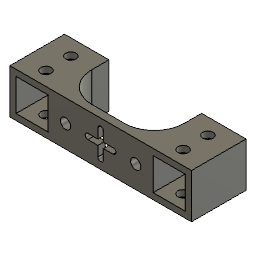
MountingBracket (Autodesk Fusion 360 design; units mm, degrees)
Autodesk Fusion 360 part; units mm, degrees
sketch "Sketch1" plane through (0, 0, 0) normal (0, 0, 1) x (1, 0, 0)
  line L0 (-1.1, 1.1) -> (-1.1, 5.1)
  arc A0 (1.1, 5.1) -> (-1.1, 5.1) centre (0, 5.1) ccw
  line L1 (1.1, 5.1) -> (1.1, 1.1)
  line L2 (-1.1, 5.1) -> (1.1, 5.1) construction
  line L3 (1.1, 1.1) -> (-1.1, 1.1) construction
  line L4 (-1.1, 1.1) -> (-1.1, -1.1) construction
  line L5 (-1.1, -1.1) -> (1.1, -1.1) construction
  line L6 (1.1, -1.1) -> (1.1, 1.1) construction
  line L7 (1.1, 1.1) -> (-1.1, -1.1) construction
  line L8 (-1.1, 1.1) -> (1.1, -1.1) construction
  line L9 (-1.1, -1.1) -> (-5.1, -1.1)
  arc A1 (-5.1, 1.1) -> (-5.1, -1.1) centre (-5.1, 0) ccw
  line L10 (-5.1, 1.1) -> (-1.1, 1.1)
  line L11 (1.1, -1.1) -> (1.1, -5.1)
  arc A2 (-1.1, -5.1) -> (1.1, -5.1) centre (0, -5.1) ccw
  line L12 (-1.1, -5.1) -> (-1.1, -1.1)
  line L13 (1.1, 1.1) -> (5.1, 1.1)
  arc A3 (5.1, -1.1) -> (5.1, 1.1) centre (5.1, 0) ccw
  line L14 (5.1, -1.1) -> (1.1, -1.1)
  line L15 (7.1, 7.1) -> (-7.1, 7.1)
  line L16 (-7.1, 7.1) -> (-7.1, -7.1)
  line L17 (-7.1, -7.1) -> (7.1, -7.1)
  line L18 (7.1, -7.1) -> (7.1, 7.1)
  line L19 (7.1, 7.1) -> (-7.1, -7.1) construction
  line L20 (-7.1, 7.1) -> (7.1, -7.1) construction
  dimension "d2" = 2.2
  dimension "d3" = 2.2
  dimension "d4" = 2.2
  dimension "d5" = 4
  dimension "d7" = 360
  dimension "d37" = 2
  constraint vertical L0
  constraint tangent L0 A0
  constraint vertical L1
  constraint horizontal L2
  constraint horizontal L3
  constraint perpendicular L3 L4
  constraint parallel L3 L5
  constraint parallel L4 L6
  constraint coincident L7 origin
  constraint coincident L8 origin
  constraint coincident L0.start L3.end
  constraint coincident L1.end L3.start
  constraint horizontal L15
  constraint perpendicular L15 L16
  constraint parallel L15 L17
  constraint parallel L16 L18
  constraint coincident L19 origin
  constraint coincident L20 origin
  constraint equal L15 L18
  measures "d2" distance of L0 L1
  measures "d3" distance of L4.end L5.end
  measures "d4" distance of L0.start L4.end
  measures "d5" distance of L2 L3
  measures "d37" distance of A3.centre L18
extrude "Extrude1" add sketch "Sketch1" along normal blind 3
sketch "Sketch2" plane through (0, 0, 0) normal (0, 0, 1) x (1, 0, 0)
  line L0 (-33.9, 6.35) -> (-21.2, 6.35) construction
  line L1 (-21.2, 6.35) -> (-21.2, -6.35) construction
  line L2 (-21.2, -6.35) -> (-33.9, -6.35) construction
  line L3 (-33.9, -6.35) -> (-33.9, 6.35) construction
  line L4 (21.2, 6.35) -> (33.9, 6.35) construction
  line L5 (33.9, 6.35) -> (33.9, -6.35) construction
  line L6 (33.9, -6.35) -> (21.2, -6.35) construction
  line L7 (21.2, -6.35) -> (21.2, 6.35) construction
  line L8 (-21.2, 0) -> (21.2, 0) construction
  line L9 (-21.1, -6.45) -> (-34, -6.45)
  line L10 (-34, -6.45) -> (-34, 6.45)
  line L11 (-34, 6.45) -> (-21.1, 6.45)
  line L12 (-21.1, 6.45) -> (-21.1, -6.45)
  line L13 (-18.6, -8.95) -> (-36.5, -8.95)
  line L14 (-36.5, -8.95) -> (-36.5, 8.95)
  line L15 (-36.5, 8.95) -> (-18.6, 8.95)
  line L16 (-18.6, 8.95) -> (-18.6, -8.95)
  line L17 (0, 2.5) -> (0, 20)
  line L18 (34, -6.45) -> (34, 6.45)
  line L19 (34, 6.45) -> (21.1, 6.45)
  line L20 (21.1, 6.45) -> (21.1, -6.45)
  line L21 (21.1, -6.45) -> (34, -6.45)
  line L22 (36.5, -8.95) -> (36.5, 8.95)
  line L23 (36.5, 8.95) -> (18.6, 8.95)
  line L24 (18.6, -8.95) -> (36.5, -8.95)
  line L25 (18.6, 8.95) -> (18.6, -8.95)
  line L26 (-18.6, -2.6) -> (-18.6, -8.95)
  line L27 (-18.6, 8.95) -> (18.6, 8.95)
  line L28 (18.6, -8.95) -> (-18.6, -8.95)
  line L29 (-7.1, 7.1) -> (-7.1, -7.1)
  line L30 (-7.1, -7.1) -> (7.1, -7.1)
  line L31 (7.1, -7.1) -> (7.1, 7.1)
  line L32 (7.1, 7.1) -> (-7.1, 7.1)
  dimension "d18" = 12.7
  dimension "d19" = 12.7
  dimension "d20" = 42.4
  dimension "d23" = -2.5
  constraint horizontal L0
  constraint vertical L1
  constraint horizontal L2
  constraint vertical L3
  constraint horizontal L4
  constraint vertical L5
  constraint horizontal L6
  constraint vertical L7
  constraint equal L0 L4
  constraint equal L3 L7
  constraint collinear L0 L4
  constraint midpoint L1 L8.start
  constraint midpoint L7 L8.end
  constraint coincident L8 origin
  constraint midpoint L8 origin
  constraint symmetric L9.start L17 L20.end
  constraint symmetric L9.end L17 L18.start
  constraint symmetric L10.end L17 L18.end
  constraint symmetric L11.end L17 L19.end
  constraint symmetric L13.start L17 L24.start
  constraint symmetric L13.end L17 L22.start
  constraint symmetric L14.end L17 L22.end
  constraint symmetric L15.end L17 L23.end
  constraint vertical L26
  measures "d18" distance of L0.start L0.end
  measures "d19" distance of L0.start L2.end
  measures "d20" distance of L1 L7
extrude "Extrude2" add sketch "Sketch2" along normal blind 3
extrude "Extrude3" add sketch "Sketch2" against normal blind 19 contours L13 L14 L15 L16 L26 | L22 L23 L24 L25
fillet "Fillet1" radius 12 2 edges at (-18.6, 0, 0) (18.6, 0, 0)
sketch "Sketch3" plane through (0, 8.95, 0) normal (0, 1, 0) x (-1, 0, 0)
  line L0 (36.5, -19) -> (36.5, 3)
  line L1 (36.5, 3) -> (-36.5, 3)
  line L2 (18.6, -12) -> (18.6, -19)
  line L3 (-36.5, -19) -> (-18.6, -19)
  circle A0 centre (-27.55, -12.6) radius 2.075
  circle A1 centre (-27.55, -2.6) radius 2.075
  line L4 (-27.55, -19) -> (-27.55, 3) construction
  line L5 (-36.5, 3) -> (-36.5, -19)
  line L6 (-18.6, -19) -> (-18.6, -12)
  line L7 (18.6, -19) -> (36.5, -19)
  line L8 (0, 1.75) -> (0, 22.5)
  circle A2 centre (27.55, -12.6) radius 2.075
  circle A3 centre (27.55, -2.6) radius 2.075
  dimension "d32" = 4.15
  dimension "d33" = 10
  dimension "d34" = 5.6
  constraint equal A0 A1
  constraint midpoint L3 L4.start
  constraint coincident A0.centre L4
  constraint coincident A1.centre L4
  constraint coincident L1 L4.end
  constraint vertical L4
  constraint symmetric A0 L8 A2
  constraint symmetric A1 L8 A3
  measures "d32" diameter of A0
  measures "d33" distance of A0.centre A1.centre
  measures "d34" distance of L1 A1.centre
extrude "Extrude4" cut sketch "Sketch3" against normal blind 17.9
sketch "Sketch4" plane through (0, 0, 3) normal (0, 0, 1) x (1, 0, 0)
  line L0 (36.5, -8.95) -> (36.5, 8.95)
  line L1 (36.5, 8.95) -> (-36.5, 8.95)
  line L2 (-36.5, 8.95) -> (-36.5, -8.95)
  line L3 (-36.5, -8.95) -> (36.5, -8.95)
  line L4 (-34, 6.45) -> (-21.1, 6.45)
  line L5 (-21.1, 6.45) -> (-21.1, -6.45)
  line L6 (-21.1, -6.45) -> (-34, -6.45)
  line L7 (-34, -6.45) -> (-34, 6.45)
  line L8 (34, -6.45) -> (21.1, -6.45)
  line L9 (21.1, -6.45) -> (21.1, 6.45)
  line L10 (21.1, 6.45) -> (34, 6.45)
  line L11 (34, 6.45) -> (34, -6.45)
  arc A0 (1.1, 5.1) -> (-1.1, 5.1) centre (0, 5.1) ccw
  line L12 (1.1, 5.1) -> (1.1, 1.1)
  line L13 (1.1, 1.1) -> (5.1, 1.1)
  arc A1 (5.1, -1.1) -> (5.1, 1.1) centre (5.1, 0) ccw
  line L14 (5.1, -1.1) -> (1.1, -1.1)
  line L15 (1.1, -1.1) -> (1.1, -5.1)
  arc A2 (-1.1, -5.1) -> (1.1, -5.1) centre (0, -5.1) ccw
  line L16 (-1.1, -5.1) -> (-1.1, -1.1)
  line L17 (-1.1, -1.1) -> (-5.1, -1.1)
  arc A3 (-5.1, 1.1) -> (-5.1, -1.1) centre (-5.1, 0) ccw
  line L18 (-5.1, 1.1) -> (-1.1, 1.1)
  line L19 (-1.1, 1.1) -> (-1.1, 5.1)
  line L20 (-21.1, 6.45) -> (-21.1, -6.45)
  line L21 (21.1, -6.45) -> (21.1, 6.45)
  line L22 (-21.1, 0) -> (21.1, 0) construction
  circle A4 centre (-14.1, 0) radius 2.075
  line L23 (0, 2.5) -> (0, 20)
  circle A5 centre (14.1, 0) radius 2.075
  dimension "d38" = 7
  dimension "d39" = 4.15
  constraint midpoint L5 L22.start
  constraint midpoint L9 L22.end
  constraint coincident L22 A4.centre
  constraint symmetric A4 L23 A5
  measures "d38" distance of L20 A4.centre
  measures "d39" diameter of A4
extrude "Extrude5" cut sketch "Sketch4" against normal blind 22 contours A4 | A5
ref_plane "WorkPlane1" through (0, 0, -6) normal (0, 0, -1) x (-1, 0, 0)
sketch "Sketch5" plane through (0, 0, -6) normal (0, 0, -1) x (-1, 0, 0)
  line L0 (-21.1, 6.45) -> (-21.1, -6.45)
  line L1 (21.1, -6.45) -> (21.1, 6.45)
  line L2 (-21.1, 0) -> (21.1, 0) construction
  circle A0 centre (-14.1, 0) radius 4.5
  line L3 (0, 1.75) -> (0, 22.5)
  circle A1 centre (14.1, 0) radius 4.5
  line L4 (-17.7, 2.7) -> (-17.7, -2.7)
  line L5 (17.7, 2.7) -> (17.7, -2.7)
  dimension "d43" = 9
  dimension "d44" = 7
  dimension "d49" = 3.6
  constraint midpoint L0 L2.start
  constraint midpoint L1 L2.end
  constraint coincident L2 A0.centre
  constraint symmetric A0 L3 A1
  constraint coincident A0 L4.start
  constraint coincident A0 L4.end
  constraint vertical L4
  constraint symmetric L3 L4.start L5.start
  constraint symmetric L3 L4.end L5.end
  measures "d43" diameter of A0
  measures "d44" distance of L0 A0.centre
  measures "d49" distance of A0.centre L4
extrude "Extrude6" cut sketch "Sketch5" along normal blind -6 and the other way blind -45.366 contours A0 L4 | A1 L5 picked at (-15.387, 1.0056) picked at (14.9987, -0.474)
equation "mounting_size = 2.2 mm"
equation "d2 = mounting_size"
equation "d3 = mounting_size"
equation "d4 = mounting_size"
equation "d21 = -tolerance_bar"
equation "tolerance_bar = 0.1 mm"
equation "d30 = 13 mm - ( 4 / 4 ) * 1 mm"
equation "tolerance_hole = 0.15 mm"
equation "d32 = 4 mm + tolerance_hole"
equation "d39 = 4 mm + tolerance_hole"
equation "d49 = ( 7 / 2 ) * 1 mm + 0.1 mm"
